Autodesk Fusion 360 part; units mm, degrees
note: some values were not read from the file. Set by a fixed rule: which sketch regions a step uses.
(part 2 of 4)
  spline S190 degree 3 poles (159.041, -110.49) (158.9881, -111.6013) (157.4271, -114.2471) (156.1835, -115.2525) knots 0 0 0 0 1 1 1 1
  spline S191 degree 3 poles (156.1835, -115.2525) (154.7283, -116.4431) (153.0085, -116.9458) (150.3892, -116.9458) knots 0 0 0 0 1 1 1 1
  spline S192 degree 3 poles (150.3892, -116.9458) (148.9604, -116.9458) (148.3519, -117.0517) (147.9285, -117.3956) knots 0 0 0 0 1 1 1 1
  line L118 (147.9285, -117.3956) -> (147.3465, -117.8719)
  line L119 (147.3465, -117.8719) -> (147.9021, -119.4594)
  spline S193 degree 3 poles (147.9021, -119.4594) (148.881, -122.211) (149.2779, -124.8304) (149.2515, -128.4552) knots 0 0 0 0 1 1 1 1
  spline S194 degree 3 poles (149.2515, -128.4552) (149.2515, -132.5298) (148.5635, -135.7048) (146.8967, -139.2502) knots 0 0 0 0 1 1 1 1
  line L120 (146.8967, -139.2502) -> (145.8648, -141.4727)
  line L121 (145.8648, -141.4727) -> (146.9496, -141.2346)
  spline S195 degree 3 poles (146.9496, -141.2346) (147.5317, -141.0758) (149.0133, -141.0229) (150.2304, -141.1023) knots 0 0 0 0 1 1 1 1
  spline S196 degree 3 poles (150.2304, -141.1023) (153.035, -141.261) (155.1781, -142.2135) (155.7338, -143.5629) knots 0 0 0 0 1 1 1 1
  spline S197 degree 3 poles (155.7338, -143.5629) (156.2365, -144.7271) (156.21, -147.8227) (155.6808, -151.2094) knots 0 0 0 0 1 1 1 1
  spline S198 degree 3 poles (155.6808, -151.2094) (155.231, -154.1462) (155.284, -154.7813) (156.0248, -154.7813) knots 0 0 0 0 1 1 1 1
  spline S199 degree 3 poles (156.0248, -154.7813) (157.136, -154.7813) (158.1944, -153.7494) (159.1469, -151.765) knots 0 0 0 0 1 1 1 1
  spline S200 degree 3 poles (159.1469, -151.765) (160.1258, -149.7013) (160.7344, -149.1192) (161.7398, -149.2779) knots 0 0 0 0 1 1 1 1
  spline S201 degree 3 poles (161.7398, -149.2779) (162.6658, -149.4102) (162.6394, -150.5479) (161.6604, -151.474) knots 0 0 0 0 1 1 1 1
  spline S202 degree 3 poles (161.6604, -151.474) (160.7873, -152.2942) (160.6021, -153.1938) (161.3165, -153.1938) knots 0 0 0 0 1 1 1 1
  spline S203 degree 3 poles (161.3165, -153.1938) (161.5546, -153.1938) (162.5071, -152.9027) (163.4067, -152.5323) knots 0 0 0 0 1 1 1 1
  spline S204 degree 3 poles (163.4067, -152.5323) (164.9677, -151.8973) (167.0315, -151.6063) (167.3754, -151.9502) knots 0 0 0 0 1 1 1 1
  spline S205 degree 3 poles (167.3754, -151.9502) (167.8252, -152.3735) (167.1108, -153.1938) (166.079, -153.4583) knots 0 0 0 0 1 1 1 1
  spline S206 degree 3 poles (166.079, -153.4583) (164.5708, -153.8288) (162.56, -154.8606) (162.7188, -155.1781) knots 0 0 0 0 1 1 1 1
  spline S207 degree 3 poles (162.7188, -155.1781) (162.7981, -155.3104) (163.0363, -155.4163) (163.2479, -155.3633) knots 0 0 0 0 1 1 1 1
  spline S208 degree 3 poles (163.2479, -155.3633) (164.9942, -154.9929) (166.661, -154.8077) (168.8835, -154.8077) knots 0 0 0 0 1 1 1 1
  spline S209 degree 3 poles (168.8835, -154.8077) (171.3971, -154.7813) (171.4765, -154.8077) (171.3971, -155.3633) knots 0 0 0 0 1 1 1 1
  spline S210 degree 3 poles (171.3971, -155.3633) (171.3177, -155.9983) (170.9473, -156.1306) (168.1427, -156.6333) knots 0 0 0 0 1 1 1 1
  spline S211 degree 3 poles (168.1427, -156.6333) (165.7615, -157.0831) (163.7771, -157.6652) (163.7771, -157.9298) knots 0 0 0 0 1 1 1 1
  spline S212 degree 3 poles (163.7771, -157.9298) (163.7771, -158.2738) (166.37, -159.0146) (169.0158, -159.4115) knots 0 0 0 0 1 1 1 1
  spline S213 degree 3 poles (169.0158, -159.4115) (171.7675, -159.8348) (171.9792, -159.9142) (171.9792, -160.5756) knots 0 0 0 0 1 1 1 1
  spline S214 degree 3 poles (171.9792, -160.5756) (171.9792, -161.7663) (171.0267, -161.925) (168.1956, -161.1048) knots 0 0 0 0 1 1 1 1
  spline S215 degree 3 poles (168.1956, -161.1048) (167.1638, -160.8138) (165.1529, -160.5227) (163.7771, -160.4433) knots 0 0 0 0 1 1 1 1
  spline S216 degree 3 poles (163.7771, -160.4433) (161.581, -160.311) (161.3165, -160.3375) (161.7398, -160.6815) knots 0 0 0 0 1 1 1 1
  spline S217 degree 3 poles (161.7398, -160.6815) (161.9779, -160.8931) (162.7981, -161.1313) (163.539, -161.2106) knots 0 0 0 0 1 1 1 1
  spline S218 degree 3 poles (163.539, -161.2106) (165.1, -161.3958) (165.6821, -161.7927) (165.5763, -162.56) knots 0 0 0 0 1 1 1 1
  spline S219 degree 3 poles (165.5763, -162.56) (165.4969, -163.0627) (165.3381, -163.1156) (164.0417, -163.0892) knots 0 0 0 0 1 1 1 1
  spline S220 degree 3 poles (164.0417, -163.0892) (163.2479, -163.0627) (161.925, -162.7981) (161.1313, -162.5071) knots 0 0 0 0 1 1 1 1
  spline S221 degree 3 poles (161.1313, -162.5071) (154.1992, -159.9406) (153.67, -159.7025) (152.4529, -158.459) knots 0 0 0 0 1 1 1 1
  spline S222 degree 3 poles (152.4529, -158.459) (151.0506, -157.0302) (150.0188, -153.4848) (150.0188, -150.0452) knots 0 0 0 0 1 1 1 1
  spline S223 degree 3 poles (150.0188, -150.0452) (150.0188, -148.8017) (149.9658, -148.6694) (149.569, -148.8546) knots 0 0 0 0 1 1 1 1
  spline S224 degree 3 poles (149.569, -148.8546) (148.6694, -149.225) (145.6531, -149.9923) (144.9388, -149.9923) knots 0 0 0 0 1 1 1 1
  spline S225 degree 3 poles (144.9388, -149.9923) (144.1979, -150.0188) (144.1979, -150.0188) (144.1979, -151.8708) knots 0 0 0 0 1 1 1 1
  spline S226 degree 3 poles (144.1979, -151.8708) (144.1979, -154.305) (143.51, -156.3158) (141.5521, -159.676) knots 0 0 0 0 1 1 1 1
  spline S227 degree 3 poles (141.5521, -159.676) (138.5888, -164.809) (137.1335, -169.201) (136.869, -173.8313) knots 0 0 0 0 1 1 1 1
  spline S228 degree 3 poles (136.869, -173.8313) (136.4985, -181.1073) (139.5677, -185.42) (147.664, -189.0183) knots 0 0 0 0 1 1 1 1
  spline S229 degree 3 poles (147.664, -189.0183) (151.13, -190.5529) (157.4271, -191.0292) (162.0044, -190.0767) knots 0 0 0 0 1 1 1 1
  spline S230 degree 3 poles (162.0044, -190.0767) (169.7038, -188.5156) (175.8685, -184.6792) (181.4777, -177.9323) knots 0 0 0 0 1 1 1 1
  line L122 (181.4777, -177.9323) -> (182.3508, -176.874)
  line L123 (182.3508, -176.874) -> (181.6629, -178.1969)
  spline S231 degree 3 poles (181.6629, -178.1969) (178.4879, -184.2029) (172.1379, -189.1242) (164.0417, -191.8494) knots 0 0 0 0 1 1 1 1
  spline S232 degree 3 poles (164.0417, -191.8494) (155.1252, -194.8392) (147.0025, -194.7863) (139.6735, -191.6906) knots 0 0 0 0 1 1 1 1
  spline S233 degree 3 poles (139.6735, -191.6906) (127.344, -186.5048) (124.5658, -178.2233) (130.0163, -163.0627) knots 0 0 0 0 1 1 1 1
  spline S234 degree 3 poles (130.0163, -163.0627) (131.2333, -159.7025) (131.4979, -156.9773) (130.8894, -153.8552) knots 0 0 0 0 1 1 1 1
  spline S235 degree 3 poles (130.8894, -153.8552) (130.3338, -150.8919) (130.0427, -150.3098) (129.0638, -149.8865) knots 0 0 0 0 1 1 1 1
  spline S236 degree 3 poles (129.0638, -149.8865) (128.5875, -149.7013) (127.6615, -149.1192) (127, -148.6165) knots 0 0 0 0 1 1 1 1
  line L124 (127, -148.6165) -> (125.8094, -147.7169)
  line L125 (125.8094, -147.7169) -> (125.8094, -150.6538)
  spline S237 degree 3 poles (125.8094, -150.6538) (125.8094, -153.4319) (125.7565, -153.6965) (124.9627, -155.3104) knots 0 0 0 0 1 1 1 1
  spline S238 degree 3 poles (124.9627, -155.3104) (123.825, -157.6388) (123.0577, -158.3002) (119.8298, -159.7025) knots 0 0 0 0 1 1 1 1
  spline S239 degree 3 poles (119.8298, -159.7025) (113.1623, -162.6394) (110.834, -163.2479) (110.0667, -162.2954) knots 0 0 0 0 1 1 1 1
  spline S240 degree 3 poles (110.0667, -162.2954) (109.564, -161.7398) (110.1196, -161.29) (111.7865, -160.8931) knots 0 0 0 0 1 1 1 1
  spline S241 degree 3 poles (111.7865, -160.8931) (112.5273, -160.7079) (113.5063, -160.311) (113.9825, -160.02) knots 0 0 0 0 1 1 1 1
  spline S242 degree 3 poles (113.9825, -160.02) (114.7233, -159.5702) (114.8027, -159.4379) (114.5117, -159.094) knots 0 0 0 0 1 1 1 1
  spline S243 degree 3 poles (114.5117, -159.094) (114.2471, -158.75) (113.7444, -158.7235) (111.6542, -158.8558) knots 0 0 0 0 1 1 1 1
  spline S244 degree 3 poles (111.6542, -158.8558) (105.1454, -159.3056) (104.0871, -159.3321) (103.3992, -159.041) knots 0 0 0 0 1 1 1 1
  spline S245 degree 3 poles (103.3992, -159.041) (102.6319, -158.75) (102.3938, -158.0356) (103.0023, -157.824) knots 0 0 0 0 1 1 1 1
  spline S246 degree 3 poles (103.0023, -157.824) (103.161, -157.771) (104.9338, -157.5858) (106.8917, -157.4535) knots 0 0 0 0 1 1 1 1
  spline S247 degree 3 poles (106.8917, -157.4535) (110.9663, -157.1625) (112.4479, -156.7921) (111.8658, -156.1835) knots 0 0 0 0 1 1 1 1
  spline S248 degree 3 poles (111.8658, -156.1835) (111.6542, -155.9983) (111.0192, -155.7602) (110.4371, -155.6808) knots 0 0 0 0 1 1 1 1
  spline S249 degree 3 poles (110.4371, -155.6808) (108.876, -155.4427) (104.5898, -154.014) (104.2458, -153.5906) knots 0 0 0 0 1 1 1 1
  spline S250 degree 3 poles (104.2458, -153.5906) (104.0606, -153.379) (104.0077, -153.0085) (104.0871, -152.7704) knots 0 0 0 0 1 1 1 1
  spline S251 degree 3 poles (104.0871, -152.7704) (104.2988, -152.2413) (105.5158, -152.3735) (109.2729, -153.3525) knots 0 0 0 0 1 1 1 1
  spline S252 degree 3 poles (109.2729, -153.3525) (112.1304, -154.0669) (112.7125, -154.1198) (112.7125, -153.6435) knots 0 0 0 0 1 1 1 1
  spline S253 degree 3 poles (112.7125, -153.6435) (112.7125, -153.1938) (111.76, -152.2942) (110.146, -151.2358) knots 0 0 0 0 1 1 1 1
  spline S254 degree 3 poles (110.146, -151.2358) (108.876, -150.4156) (108.4527, -149.6748) (108.9554, -149.1721) knots 0 0 0 0 1 1 1 1
  spline S255 degree 3 poles (108.9554, -149.1721) (109.4317, -148.6958) (110.781, -149.225) (112.6067, -150.5744) knots 0 0 0 0 1 1 1 1
  spline S256 degree 3 poles (112.6067, -150.5744) (113.5856, -151.2887) (114.4852, -151.8708) (114.591, -151.8708) knots 0 0 0 0 1 1 1 1
  spline S257 degree 3 poles (114.591, -151.8708) (114.9879, -151.8708) (114.8556, -150.839) (114.3, -149.7542) knots 0 0 0 0 1 1 1 1
  spline S258 degree 3 poles (114.3, -149.7542) (113.6121, -148.4048) (113.6121, -147.2142) (114.2735, -147.029) knots 0 0 0 0 1 1 1 1
  spline S259 degree 3 poles (114.2735, -147.029) (114.9879, -146.8438) (115.8875, -147.5317) (115.8875, -148.246) knots 0 0 0 0 1 1 1 1
  spline S260 degree 3 poles (115.8875, -148.246) (115.8875, -149.3044) (118.2158, -152.2413) (119.38, -152.6381) knots 0 0 0 0 1 1 1 1
  spline S261 degree 3 poles (119.38, -152.6381) (120.2002, -152.9292) (120.9146, -152.7704) (120.9146, -152.2942) knots 0 0 0 0 1 1 1 1
  spline S262 degree 3 poles (120.9146, -152.2942) (120.9146, -152.1354) (120.6765, -151.1035) (120.3854, -150.0188) knots 0 0 0 0 1 1 1 1
  spline S263 degree 3 poles (120.3854, -150.0188) (119.4858, -146.6056) (119.8563, -143.3248) (121.3115, -141.605) knots 0 0 0 0 1 1 1 1
  spline S264 degree 3 poles (121.3115, -141.605) (122.1581, -140.5996) (122.9783, -140.4408) (125.5448, -140.9171) knots 0 0 0 0 1 1 1 1
  spline S265 degree 3 poles (125.5448, -140.9171) (126.709, -141.1023) (127.926, -141.2875) (128.2435, -141.2875) knots 0 0 0 0 1 1 1 1
  line L126 (128.2435, -141.2875) -> (128.8256, -141.2875)
  line L127 (128.8256, -141.2875) -> (128.0054, -139.0915)
  spline S266 degree 3 poles (128.0054, -139.0915) (125.3596, -132.08) (124.5129, -127.8202) (124.6981, -122.5021) knots 0 0 0 0 1 1 1 1
  spline S267 degree 3 poles (124.6981, -122.5021) (124.8304, -119.1948) (125.1479, -117.5015) (126.0475, -115.3319) knots 0 0 0 0 1 1 1 1
  spline S268 degree 3 poles (126.0475, -115.3319) (126.3385, -114.6704) (124.9363, -114.3) (122.2375, -114.3) knots 0 0 0 0 1 1 1 1
  spline S269 degree 3 poles (122.2375, -114.3) (120.1473, -114.3) (119.8563, -114.2206) (118.6392, -113.4798) knots 0 0 0 0 1 1 1 1
  spline S270 degree 3 poles (118.6392, -113.4798) (117.9248, -113.03) (116.9988, -112.3421) (116.5754, -111.9452) knots 0 0 0 0 1 1 1 1
  spline S271 degree 3 poles (116.5754, -111.9452) (115.7817, -111.2308) (114.5646, -108.929) (114.5646, -108.1881) knots 0 0 0 0 1 1 1 1
  spline S272 degree 3 poles (114.5646, -108.1881) (114.5646, -107.7383) (113.321, -106.4948) (112.051, -105.6746) knots 0 0 0 0 1 1 1 1
  spline S273 degree 3 poles (112.051, -105.6746) (111.7071, -105.4365) (110.9398, -105.1983) (110.3313, -105.1454) knots 0 0 0 0 1 1 1 1
  spline S274 degree 3 poles (110.3313, -105.1454) (108.8496, -105.0131) (106.5742, -103.8225) (106.68, -103.2404) knots 0 0 0 0 1 1 1 1
  spline S275 degree 3 poles (106.68, -103.2404) (106.7858, -102.7906) (107.4473, -102.7112) (109.0083, -102.9494) knots 0 0 0 0 1 1 1 1
  spline S276 degree 3 poles (109.0083, -102.9494) (109.511, -103.0288) (109.6963, -102.9229) (109.7492, -102.526) knots 0 0 0 0 1 1 1 1
  spline S277 degree 3 poles (109.7492, -102.526) (109.8021, -102.1556) (108.9819, -101.1502) (107.1563, -99.2981) knots 0 0 0 0 1 1 1 1
  spline S278 degree 3 poles (107.1563, -99.2981) (105.701, -97.8165) (104.5104, -96.4671) (104.5104, -96.3083) knots 0 0 0 0 1 1 1 1
  spline S279 degree 3 poles (104.5104, -96.3083) (104.5104, -95.8585) (105.754, -95.6998) (106.7329, -96.0438) knots 0 0 0 0 1 1 1 1
  spline S280 degree 3 poles (106.7329, -96.0438) (107.315, -96.229) (108.0558, -96.8375) (108.6644, -97.5783) knots 0 0 0 0 1 1 1 1
  spline S281 degree 3 poles (108.6644, -97.5783) (109.22, -98.2662) (109.8021, -98.9012) (109.9344, -99.0071) knots 0 0 0 0 1 1 1 1
  spline S282 degree 3 poles (109.9344, -99.0071) (110.834, -99.6685) (110.8075, -98.6102) (109.8815, -96.7317) knots 0 0 0 0 1 1 1 1
  spline S283 degree 3 poles (109.8815, -96.7317) (109.1671, -95.2235) (109.1935, -94.4563) (110.0138, -94.4563) knots 0 0 0 0 1 1 1 1
  spline S284 degree 3 poles (110.0138, -94.4563) (110.7017, -94.4563) (111.4954, -95.4087) (112.2892, -97.155) knots 0 0 0 0 1 1 1 1
  spline S285 degree 3 poles (112.2892, -97.155) (113.321, -99.5362) (114.0354, -99.0865) (114.0354, -96.0967) knots 0 0 0 0 1 1 1 1
  spline S286 degree 3 poles (114.0354, -96.0967) (114.0354, -94.959) (114.1677, -94.5621) (114.7233, -94.0065) knots 0 0 0 0 1 1 1 1
  spline S287 degree 3 poles (114.7233, -94.0065) (115.3319, -93.3979) (115.4377, -93.3715) (115.8081, -93.7154) knots 0 0 0 0 1 1 1 1
  spline S288 degree 3 poles (115.8081, -93.7154) (116.1256, -94.0594) (116.1521, -94.324) (115.914, -95.1442) knots 0 0 0 0 1 1 1 1
  spline S289 degree 3 poles (115.914, -95.1442) (115.5435, -96.4671) (115.5435, -98.5837) (115.8875, -99.2452) knots 0 0 0 0 1 1 1 1
  spline S290 degree 3 poles (115.8875, -99.2452) (116.3902, -100.1712) (117.1575, -99.8538) (117.8719, -98.425) knots 0 0 0 0 1 1 1 1
  spline S291 degree 3 poles (117.8719, -98.425) (118.3481, -97.4725) (118.6921, -97.1021) (119.089, -97.1021) knots 0 0 0 0 1 1 1 1
  spline S292 degree 3 poles (119.089, -97.1021) (119.7504, -97.1021) (119.671, -97.3931) (118.3481, -100.3829) knots 0 0 0 0 1 1 1 1
  spline S293 degree 3 poles (118.3481, -100.3829) (117.3427, -102.6054) (117.0517, -104.0606) (117.3163, -105.1719) knots 0 0 0 0 1 1 1 1
  spline S294 degree 3 poles (117.3163, -105.1719) (117.5015, -105.9392) (118.9302, -107.5796) (120.3854, -108.7438) knots 0 0 0 0 1 1 1 1
  line L128 (120.3854, -108.7438) -> (121.3644, -109.511)
  line L129 (121.3644, -109.511) -> (123.4281, -108.8496)
  spline S295 degree 3 poles (123.4281, -108.8496) (124.751, -108.4262) (126.1533, -108.1881) (127.3704, -108.1617) knots 0 0 0 0 1 1 1 1
  line L130 (127.3704, -108.1617) -> (129.249, -108.1352)
  line L131 (129.249, -108.1352) -> (130.4131, -106.68)
  spline S296 degree 3 poles (130.4131, -106.68) (131.736, -105.0131) (132.1858, -103.7167) (131.7625, -102.9229) knots 0 0 0 0 1 1 1 1
  spline S297 degree 3 poles (131.7625, -102.9229) (131.6038, -102.6319) (131.3921, -102.3938) (131.2598, -102.3938) knots 0 0 0 0 1 1 1 1
  spline S298 degree 3 poles (131.2598, -102.3938) (130.7571, -102.3938) (129.1167, -100.3829) (128.7463, -99.2717) knots 0 0 0 0 1 1 1 1
  spline S299 degree 3 poles (128.7463, -99.2717) (128.27, -97.8958) (128.1906, -94.0594) (128.5875, -92.5777) knots 0 0 0 0 1 1 1 1
  spline S300 degree 3 poles (128.5875, -92.5777) (128.7463, -92.0485) (129.1431, -91.2019) (129.5135, -90.7256) knots 0 0 0 0 1 1 1 1
  spline S301 degree 3 poles (129.5135, -90.7256) (129.8575, -90.2229) (130.3338, -89.4292) (130.5454, -88.9794) knots 0 0 0 0 1 1 1 1
  spline S302 degree 3 poles (130.5454, -88.9794) (130.7571, -88.5031) (131.2863, -87.6035) (131.7096, -86.995) knots 0 0 0 0 1 1 1 1
  spline S303 degree 3 poles (131.7096, -86.995) (132.1329, -86.36) (132.8473, -85.09) (133.2706, -84.1375) knots 0 0 0 0 1 1 1 1
  spline S304 degree 3 poles (133.2706, -84.1375) (134.1173, -82.259) (135.4138, -80.645) (136.6573, -79.8512) knots 0 0 0 0 1 1 1 1
  spline S305 degree 3 poles (136.6573, -79.8512) (137.7156, -79.1633) (140.679, -79.3221) (142.24, -80.1158) knots 0 0 0 0 1 1 1 1
  spline S306 degree 3 poles (215.6354, -67.7598) (211.0581, -70.9612) (207.2217, -73.66) (207.0894, -73.7923) knots 0 0 0 0 1 1 1 1
  spline S307 degree 3 poles (207.0894, -73.7923) (206.8248, -74.0569) (213.6775, -84.164) (216.8525, -88.265) knots 0 0 0 0 1 1 1 1
  spline S308 degree 3 poles (216.8525, -88.265) (219.0221, -91.0696) (221.4298, -93.2127) (223.5729, -94.271) knots 0 0 0 0 1 1 1 1
  spline S309 degree 3 poles (223.5729, -94.271) (224.9752, -94.959) (225.6102, -95.1177) (227.039, -95.1177) knots 0 0 0 0 1 1 1 1
  spline S310 degree 3 poles (227.039, -95.1177) (228.5471, -95.1177) (229.0498, -94.9854) (230.796, -94.0858) knots 0 0 0 0 1 1 1 1
  spline S311 degree 3 poles (230.796, -94.0858) (233.389, -92.7894) (235.9025, -90.514) (236.6963, -88.7677) knots 0 0 0 0 1 1 1 1
  spline S312 degree 3 poles (236.6963, -88.7677) (237.9398, -86.1219) (237.3577, -82.4442) (235.0294, -78.0521) knots 0 0 0 0 1 1 1 1
  spline S313 degree 3 poles (235.0294, -78.0521) (233.8917, -75.909) (224.3931, -61.886) (224.1021, -61.939) knots 0 0 0 0 1 1 1 1
  spline S314 degree 3 poles (224.1021, -61.939) (224.0227, -61.939) (220.2127, -64.5848) (215.6354, -67.7598) knots 0 0 0 0 1 1 1 1
  spline S315 degree 3 poles (227.0654, -75.0358) (231.0606, -80.8567) (230.9283, -83.82) (226.5627, -86.069) knots 0 0 0 0 1 1 1 1
  spline S316 degree 3 poles (226.5627, -86.069) (224.6842, -87.0479) (222.2765, -86.3335) (220.3715, -84.2433) knots 0 0 0 0 1 1 1 1
  spline S317 degree 3 poles (220.3715, -84.2433) (219.3131, -83.0792) (216.1381, -78.5283) (216.2175, -78.2638) knots 0 0 0 0 1 1 1 1
  spline S318 degree 3 poles (216.2175, -78.2638) (216.3498, -77.8933) (224.7106, -72.2048) (225.0017, -72.3106) knots 0 0 0 0 1 1 1 1
  spline S319 degree 3 poles (225.0017, -72.3106) (225.134, -72.3635) (226.06, -73.5806) (227.0654, -75.0358) knots 0 0 0 0 1 1 1 1
  spline S320 degree 3 poles (57.5469, -81.1212) (55.245, -84.6931) (53.2606, -87.6565) (53.1283, -87.7358) knots 0 0 0 0 1 1 1 1
  spline S321 degree 3 poles (53.1283, -87.7358) (52.996, -87.8152) (49.9269, -85.9367) (46.2756, -83.5819) knots 0 0 0 0 1 1 1 1
  spline S322 degree 3 poles (46.2756, -83.5819) (42.6508, -81.2271) (39.5552, -79.4015) (39.4494, -79.5337) knots 0 0 0 0 1 1 1 1
  spline S323 degree 3 poles (39.4494, -79.5337) (38.4969, -80.6715) (34.8985, -86.5981) (35.0838, -86.7833) knots 0 0 0 0 1 1 1 1
  spline S324 degree 3 poles (35.0838, -86.7833) (35.4542, -87.1273) (52.1494, -97.9223) (52.414, -97.9752) knots 0 0 0 0 1 1 1 1
  spline S325 degree 3 poles (52.414, -97.9752) (52.5727, -98.0017) (55.6948, -93.3979) (59.3725, -87.7094) knots 0 0 0 0 1 1 1 1
  line L132 (59.3725, -87.7094) -> (66.0929, -77.3906)
  line L133 (66.0929, -77.3906) -> (64.1879, -76.2)
  spline S326 degree 3 poles (64.1879, -76.2) (63.156, -75.5385) (62.1771, -74.9035) (62.0183, -74.7977) knots 0 0 0 0 1 1 1 1
  spline S327 degree 3 poles (62.0183, -74.7977) (61.8596, -74.7183) (60.034, -77.2583) (57.5469, -81.1212) knots 0 0 0 0 1 1 1 1
  spline S328 degree 3 poles (188.7538, -117.184) (186.9546, -118.0042) (186.2667, -120.2002) (187.325, -121.8935) knots 0 0 0 0 1 1 1 1
  spline S329 degree 3 poles (187.325, -121.8935) (188.7538, -124.2483) (192.2727, -124.0102) (193.331, -121.5231) knots 0 0 0 0 1 1 1 1
  spline S330 degree 3 poles (193.331, -121.5231) (194.0719, -119.6975) (193.2781, -117.8454) (191.3731, -117.0517) knots 0 0 0 0 1 1 1 1
  spline S331 degree 3 poles (191.3731, -117.0517) (190.2883, -116.5754) (190.0502, -116.6019) (188.7538, -117.184) knots 0 0 0 0 1 1 1 1
  spline S332 degree 3 poles (81.3329, -117.9777) (80.2217, -118.4804) (79.375, -119.7504) (79.375, -120.8881) knots 0 0 0 0 1 1 1 1
  spline S333 degree 3 poles (79.375, -120.8881) (79.375, -122.6608) (81.0154, -124.3542) (82.7617, -124.3542) knots 0 0 0 0 1 1 1 1
  spline S334 degree 3 poles (82.7617, -124.3542) (86.3865, -124.3542) (87.5506, -119.4594) (84.2963, -117.9777) knots 0 0 0 0 1 1 1 1
  spline S335 degree 3 poles (84.2963, -117.9777) (83.6877, -117.7131) (83.0263, -117.475) (82.8146, -117.475) knots 0 0 0 0 1 1 1 1
  spline S336 degree 3 poles (82.8146, -117.475) (82.6029, -117.475) (81.9415, -117.7131) (81.3329, -117.9777) knots 0 0 0 0 1 1 1 1
  spline S337 degree 3 poles (200.3954, -129.9104) (200.1044, -130.0163) (199.5223, -130.4925) (199.1519, -130.9688) knots 0 0 0 0 1 1 1 1
  spline S338 degree 3 poles (199.1519, -130.9688) (197.776, -132.5827) (198.3317, -135.1227) (200.2896, -136.1281) knots 0 0 0 0 1 1 1 1
  spline S339 degree 3 poles (200.2896, -136.1281) (202.5121, -137.2658) (205.0521, -135.6254) (205.0521, -133.0854) knots 0 0 0 0 1 1 1 1
  spline S340 degree 3 poles (205.0521, -133.0854) (205.0521, -130.6513) (202.6444, -128.9844) (200.3954, -129.9104) knots 0 0 0 0 1 1 1 1
  spline S341 degree 3 poles (92.366, -132.715) (91.1754, -133.7204) (90.8579, -135.1492) (91.5194, -136.6308) knots 0 0 0 0 1 1 1 1
  spline S342 degree 3 poles (91.5194, -136.6308) (92.9746, -139.9381) (97.8958, -138.9592) (97.8958, -135.3344) knots 0 0 0 0 1 1 1 1
  spline S343 degree 3 poles (97.8958, -135.3344) (97.8958, -133.2706) (96.5465, -132.0271) (94.3504, -132.0271) knots 0 0 0 0 1 1 1 1
  spline S344 degree 3 poles (94.3504, -132.0271) (93.4773, -132.0271) (92.9746, -132.1858) (92.366, -132.715) knots 0 0 0 0 1 1 1 1
  spline S345 degree 3 poles (180.049, -136.9748) (178.5144, -137.3717) (177.5354, -138.7475) (177.5354, -140.4938) knots 0 0 0 0 1 1 1 1
  spline S346 degree 3 poles (177.5354, -140.4938) (177.5354, -142.0019) (178.8054, -143.3777) (180.3665, -143.5894) knots 0 0 0 0 1 1 1 1
  spline S347 degree 3 poles (180.3665, -143.5894) (182.4038, -143.854) (183.9119, -142.7427) (184.2558, -140.7583) knots 0 0 0 0 1 1 1 1
  spline S348 degree 3 poles (184.2558, -140.7583) (184.6527, -138.5888) (182.2185, -136.4192) (180.049, -136.9748) knots 0 0 0 0 1 1 1 1
  spline S349 degree 3 poles (71.411, -140.2027) (70.5379, -141.0758) (70.3792, -141.3933) (70.3792, -142.3723) knots 0 0 0 0 1 1 1 1
  spline S350 degree 3 poles (70.3792, -142.3723) (70.3792, -145.4679) (73.6071, -147.0554) (75.909, -145.0975) knots 0 0 0 0 1 1 1 1
  spline S351 degree 3 poles (75.909, -145.0975) (77.2319, -144.0127) (77.4435, -142.2929) (76.491, -140.5202) knots 0 0 0 0 1 1 1 1
  spline S352 degree 3 poles (76.491, -140.5202) (76.0677, -139.7529) (74.8242, -139.1708) (73.5277, -139.1708) knots 0 0 0 0 1 1 1 1
  spline S353 degree 3 poles (73.5277, -139.1708) (72.6017, -139.1708) (72.2577, -139.3296) (71.411, -140.2027) knots 0 0 0 0 1 1 1 1
  spline S354 degree 3 poles (190.6588, -151.8973) (187.9865, -153.9875) (189.2829, -157.9563) (192.6167, -157.9563) knots 0 0 0 0 1 1 1 1
  spline S355 degree 3 poles (192.6167, -157.9563) (194.019, -157.9563) (195.0244, -157.3477) (195.6594, -156.1042) knots 0 0 0 0 1 1 1 1
  spline S356 degree 3 poles (195.6594, -156.1042) (196.7971, -153.8817) (195.1567, -151.3417) (192.6167, -151.3417) knots 0 0 0 0 1 1 1 1
  spline S357 degree 3 poles (192.6167, -151.3417) (191.7435, -151.3417) (191.1615, -151.5004) (190.6588, -151.8973) knots 0 0 0 0 1 1 1 1
  spline S358 degree 3 poles (83.1056, -152.7969) (82.0473, -153.7229) (81.5975, -155.0723) (81.9944, -156.3423) knots 0 0 0 0 1 1 1 1
  spline S359 degree 3 poles (81.9944, -156.3423) (82.4442, -157.8504) (83.3438, -158.5648) (85.0371, -158.6971) knots 0 0 0 0 1 1 1 1
  spline S360 degree 3 poles (85.0371, -158.6971) (86.36, -158.8029) (86.5188, -158.75) (87.4713, -157.8769) knots 0 0 0 0 1 1 1 1
  spline S361 degree 3 poles (87.4713, -157.8769) (88.4238, -157.0038) (88.5031, -156.845) (88.5031, -155.4427) knots 0 0 0 0 1 1 1 1
  spline S362 degree 3 poles (88.5031, -155.4427) (88.5031, -154.0404) (88.4238, -153.8817) (87.5242, -153.035) knots 0 0 0 0 1 1 1 1
  spline S363 degree 3 poles (87.5242, -153.035) (86.6775, -152.2677) (86.3335, -152.1354) (85.2223, -152.1354) knots 0 0 0 0 1 1 1 1
  spline S364 degree 3 poles (85.2223, -152.1354) (84.2169, -152.1354) (83.7406, -152.2942) (83.1056, -152.7969) knots 0 0 0 0 1 1 1 1
  spline S365 degree 3 poles (34.1048, -156.501) (29.8185, -157.6917) (26.1673, -158.7235) (26.035, -158.7765) knots 0 0 0 0 1 1 1 1
  spline S366 degree 3 poles (26.035, -158.7765) (25.8233, -158.8558) (30.9563, -178.435) (31.2738, -178.7525) knots 0 0 0 0 1 1 1 1
  spline S367 degree 3 poles (31.2738, -178.7525) (31.3796, -178.8319) (34.9515, -177.8529) (35.1102, -177.6942) knots 0 0 0 0 1 1 1 1
  spline S368 degree 3 poles (35.1102, -177.6942) (35.1631, -177.6413) (34.4223, -174.7308) (33.4698, -171.1854) knots 0 0 0 0 1 1 1 1
  spline S369 degree 3 poles (33.4698, -171.1854) (32.4908, -167.6665) (31.75, -164.7296) (31.8294, -164.6767) knots 0 0 0 0 1 1 1 1
  spline S370 degree 3 poles (31.8294, -164.6767) (31.9088, -164.5973) (32.4908, -164.3592) (33.1523, -164.174) knots 0 0 0 0 1 1 1 1
  line L134 (33.1523, -164.174) -> (34.3694, -163.8035)
  line L135 (34.3694, -163.8035) -> (34.7663, -165.1794)
  spline S371 degree 3 poles (34.7663, -165.1794) (34.9779, -165.9467) (35.5865, -168.1692) (36.1421, -170.1271) knots 0 0 0 0 1 1 1 1
  spline S372 degree 3 poles (36.1421, -170.1271) (36.6713, -172.085) (37.2004, -173.8048) (37.3063, -173.9106) knots 0 0 0 0 1 1 1 1
  spline S373 degree 3 poles (37.3063, -173.9106) (37.4915, -174.1223) (39.6081, -173.646) (40.0315, -173.3021) knots 0 0 0 0 1 1 1 1
  spline S374 degree 3 poles (40.0315, -173.3021) (40.1638, -173.1962) (39.6346, -170.8679) (38.8938, -168.1427) knots 0 0 0 0 1 1 1 1
  spline S375 degree 3 poles (38.8938, -168.1427) (38.1529, -165.4175) (37.5973, -163.1421) (37.6502, -163.0627) knots 0 0 0 0 1 1 1 1
  spline S376 degree 3 poles (37.6502, -163.0627) (37.7296, -163.0098) (38.3381, -162.7717) (38.9996, -162.5865) knots 0 0 0 0 1 1 1 1
  spline S377 degree 3 poles (38.9996, -162.5865) (39.9521, -162.2954) (40.2696, -162.269) (40.349, -162.5335) knots 0 0 0 0 1 1 1 1
  spline S378 degree 3 poles (40.349, -162.5335) (40.4019, -162.7188) (41.1427, -165.3381) (41.9629, -168.4073) knots 0 0 0 0 1 1 1 1
  spline S379 degree 3 poles (41.9629, -168.4073) (42.7831, -171.45) (43.5504, -174.0694) (43.6563, -174.1752) knots 0 0 0 0 1 1 1 1
  spline S380 degree 3 poles (43.6563, -174.1752) (43.9473, -174.5192) (47.4927, -173.4344) (47.4663, -173.011) knots 0 0 0 0 1 1 1 1
  spline S381 degree 3 poles (47.4663, -173.011) (47.4398, -172.6406) (43.8415, -159.5438) (42.836, -156.0248) knots 0 0 0 0 1 1 1 1
  spline S382 degree 3 poles (42.836, -156.0248) (42.545, -155.0458) (42.2275, -154.2521) (42.1217, -154.2785) knots 0 0 0 0 1 1 1 1
  spline S383 degree 3 poles (42.1217, -154.2785) (42.0158, -154.305) (38.4175, -155.284) (34.1048, -156.501) knots 0 0 0 0 1 1 1 1
  spline S384 degree 3 poles (236.0083, -155.2046) (232.7804, -156.5804) (230.1346, -162.2425) (230.0817, -167.8781) knots 0 0 0 0 1 1 1 1
  spline S385 degree 3 poles (230.0817, -167.8781) (230.0552, -170.3388) (230.1081, -170.6298) (230.8225, -171.9262) knots 0 0 0 0 1 1 1 1
  spline S386 degree 3 poles (230.8225, -171.9262) (232.119, -174.2281) (234.1298, -175.3923) (236.0083, -174.8896) knots 0 0 0 0 1 1 1 1
  spline S387 degree 3 poles (236.0083, -174.8896) (237.8869, -174.3869) (239.2892, -172.2438) (241.1677, -166.9521) knots 0 0 0 0 1 1 1 1
  spline S388 degree 3 poles (241.1677, -166.9521) (242.5171, -163.1421) (242.861, -162.7717) (243.5754, -164.4385) knots 0 0 0 0 1 1 1 1
  spline S389 degree 3 poles (243.5754, -164.4385) (244.1046, -165.7085) (243.6813, -167.296) (242.4906, -168.5396) knots 0 0 0 0 1 1 1 1
  spline S390 degree 3 poles (242.4906, -168.5396) (242.0144, -169.0423) (241.5646, -169.7567) (241.4588, -170.1271) knots 0 0 0 0 1 1 1 1
  spline S391 degree 3 poles (241.4588, -170.1271) (241.3794, -170.4975) (240.956, -172.0585) (240.5327, -173.6196) knots 0 0 0 0 1 1 1 1
  line L136 (240.5327, -173.6196) -> (239.7654, -176.4771)
  line L137 (239.7654, -176.4771) -> (240.8502, -176.3183)
  spline S392 degree 3 poles (240.8502, -176.3183) (244.5015, -175.7363) (246.8827, -172.7465) (248.2056, -167.0315) knots 0 0 0 0 1 1 1 1
  spline S393 degree 3 poles (248.2056, -167.0315) (249.3169, -162.1896) (248.576, -158.75) (246.036, -156.9244) knots 0 0 0 0 1 1 1 1
  spline S394 degree 3 poles (246.036, -156.9244) (242.57, -154.3844) (240.1094, -156.5275) (237.3313, -164.4915) knots 0 0 0 0 1 1 1 1
  spline S395 degree 3 poles (237.3313, -164.4915) (236.3523, -167.2696) (235.929, -167.8252) (235.3469, -167.0579) knots 0 0 0 0 1 1 1 1
  spline S396 degree 3 poles (235.3469, -167.0579) (234.5002, -165.9467) (235.0823, -163.2744) (236.3523, -162.2954) knots 0 0 0 0 1 1 1 1
  spline S397 degree 3 poles (236.3523, -162.2954) (236.8815, -161.8985) (237.199, -161.1313) (237.8604, -158.75) knots 0 0 0 0 1 1 1 1
  spline S398 degree 3 poles (237.8604, -158.75) (238.3102, -157.0831) (238.7335, -155.4956) (238.8129, -155.231) knots 0 0 0 0 1 1 1 1
  spline S399 degree 3 poles (238.8129, -155.231) (238.9188, -154.8606) (238.7865, -154.7813) (237.9398, -154.7813) knots 0 0 0 0 1 1 1 1
  spline S400 degree 3 poles (237.9398, -154.7813) (237.3842, -154.8077) (236.511, -154.9929) (236.0083, -155.2046) knots 0 0 0 0 1 1 1 1
  spline S401 degree 3 poles (42.5979, -182.4567) (38.735, -184.7056) (35.4542, -186.6371) (35.269, -186.7429) knots 0 0 0 0 1 1 1 1
  spline S402 degree 3 poles (35.269, -186.7429) (35.0573, -186.8752) (36.4596, -189.5475) (39.8463, -195.3948) knots 0 0 0 0 1 1 1 1
  spline S403 degree 3 poles (39.8463, -195.3948) (42.545, -200.0515) (44.8469, -203.9673) (44.9527, -204.0731) knots 0 0 0 0 1 1 1 1
  spline S404 degree 3 poles (44.9527, -204.0731) (45.0585, -204.179) (45.9317, -203.8085) (46.8842, -203.2529) knots 0 0 0 0 1 1 1 1
  line L138 (46.8842, -203.2529) -> (48.6304, -202.2475)
  line L139 (48.6304, -202.2475) -> (45.376, -196.6383)
  line L140 (45.376, -196.6383) -> (42.1217, -191.0292)
  line L141 (42.1217, -191.0292) -> (42.9419, -190.5265)
  spline S405 degree 3 poles (42.9419, -190.5265) (43.4181, -190.2619) (45.6935, -188.939) (48.0219, -187.5896) knots 0 0 0 0 1 1 1 1
  spline S406 degree 3 poles (48.0219, -187.5896) (50.3502, -186.2402) (52.5198, -184.9967) (52.8373, -184.785) knots 0 0 0 0 1 1 1 1
  spline S407 degree 3 poles (52.8373, -184.785) (53.3929, -184.441) (53.3929, -184.4146) (51.6467, -181.3719) knots 0 0 0 0 1 1 1 1
  spline S408 degree 3 poles (51.6467, -181.3719) (50.6677, -179.705) (49.821, -178.3292) (49.7417, -178.3556) knots 0 0 0 0 1 1 1 1
  spline S409 degree 3 poles (49.7417, -178.3556) (49.6623, -178.3556) (46.4608, -180.2077) (42.5979, -182.4567) knots 0 0 0 0 1 1 1 1
  spline S410 degree 3 poles (228.0708, -179.7315) (226.3246, -180.2077) (225.1604, -181.0279) (223.3613, -182.9594) knots 0 0 0 0 1 1 1 1
  spline S411 degree 3 poles (223.3613, -182.9594) (221.3769, -185.076) (219.7365, -187.8277) (218.731, -190.7381) knots 0 0 0 0 1 1 1 1
  spline S412 degree 3 poles (218.731, -190.7381) (218.0696, -192.6696) (217.9638, -193.2781) (218.0696, -194.9715) knots 0 0 0 0 1 1 1 1
  spline S413 degree 3 poles (218.0696, -194.9715) (218.149, -196.2944) (218.3871, -197.3527) (218.7575, -198.0406) knots 0 0 0 0 1 1 1 1
  spline S414 degree 3 poles (218.7575, -198.0406) (219.9746, -200.4219) (223.0967, -202.5121) (225.9013, -202.856) knots 0 0 0 0 1 1 1 1
  spline S415 degree 3 poles (225.9013, -202.856) (229.4467, -203.2794) (233.1244, -200.6865) (236.0877, -195.6594) knots 0 0 0 0 1 1 1 1
  spline S416 degree 3 poles (236.0877, -195.6594) (239.051, -190.6058) (239.4479, -185.8963) (237.1196, -183.1181) knots 0 0 0 0 1 1 1 1
  line L142 (237.1196, -183.1181) -> (236.4052, -182.245)
  line L143 (236.4052, -182.245) -> (234.5002, -185.4994)
  spline S417 degree 3 poles (234.5002, -185.4994) (232.9127, -188.2246) (232.6481, -188.8331) (232.8598, -189.3623) knots 0 0 0 0 1 1 1 1
  spline S418 degree 3 poles (232.8598, -189.3623) (233.6006, -191.3202) (232.066, -194.5217) (229.87, -195.6858) knots 0 0 0 0 1 1 1 1
  spline S419 degree 3 poles (229.87, -195.6858) (228.0444, -196.6383) (225.3456, -195.7388) (224.2079, -193.7808) knots 0 0 0 0 1 1 1 1
  spline S420 degree 3 poles (224.2079, -193.7808) (223.4142, -192.4315) (223.4142, -191.2673) (224.2079, -189.574) knots 0 0 0 0 1 1 1 1
  spline S421 degree 3 poles (224.2079, -189.574) (224.9752, -187.96) (226.0865, -186.8752) (227.4358, -186.399) knots 0 0 0 0 1 1 1 1
  spline S422 degree 3 poles (227.4358, -186.399) (228.3619, -186.1079) (228.6529, -185.7375) (230.2933, -182.9858) knots 0 0 0 0 1 1 1 1
  spline S423 degree 3 poles (230.2933, -182.9858) (231.2988, -181.2925) (232.0396, -179.8373) (231.9867, -179.7579) knots 0 0 0 0 1 1 1 1
  spline S424 degree 3 poles (231.9867, -179.7579) (231.6692, -179.4404) (229.1556, -179.414) (228.0708, -179.7315) knots 0 0 0 0 1 1 1 1
  line L144 (56.224, -204.8933) -> (50.1385, -210.7935)
  line L145 (50.1385, -210.7935) -> (57.4146, -218.2548)
  line L146 (57.4146, -218.2548) -> (64.6642, -225.716)
  line L147 (64.6642, -225.716) -> (66.0665, -224.3138)
  spline S425 degree 3 poles (66.0665, -224.3138) (66.8338, -223.5465) (67.4688, -222.8321) (67.4688, -222.6733) knots 0 0 0 0 1 1 1 1
  spline S426 degree 3 poles (67.4688, -222.6733) (67.4688, -222.541) (65.3785, -220.345) (62.8385, -217.7785) knots 0 0 0 0 1 1 1 1
  line L148 (62.8385, -217.7785) -> (58.2083, -213.0954)
  line L149 (58.2083, -213.0954) -> (59.2138, -212.1165)
  line L150 (59.2138, -212.1165) -> (60.1927, -211.1375)
  line L151 (60.1927, -211.1375) -> (63.9498, -214.8946)
  line L152 (63.9498, -214.8946) -> (67.7333, -218.6781)
  line L153 (67.7333, -218.6781) -> (68.8446, -217.5404)
  line L154 (68.8446, -217.5404) -> (69.9823, -216.4292)
  line L155 (69.9823, -216.4292) -> (66.1988, -212.6456)
  line L156 (66.1988, -212.6456) -> (62.4417, -208.8621)
  line L157 (62.4417, -208.8621) -> (63.4735, -207.8567)
  line L158 (63.4735, -207.8567) -> (64.5054, -206.8513)
  line L159 (64.5054, -206.8513) -> (68.7917, -211.2433)
  spline S427 degree 3 poles (68.7917, -211.2433) (71.1729, -213.651) (73.2367, -215.6354) (73.3954, -215.6354) knots 0 0 0 0 1 1 1 1
  spline S428 degree 3 poles (73.3954, -215.6354) (73.5806, -215.6354) (74.295, -215.0533) (75.0094, -214.3125) knots 0 0 0 0 1 1 1 1
  line L160 (75.0094, -214.3125) -> (76.3058, -212.9896)
  line L161 (76.3058, -212.9896) -> (75.274, -211.8783)
  spline S429 degree 3 poles (75.274, -211.8783) (73.3425, -209.7881) (62.574, -198.9667) (62.4417, -198.9667) knots 0 0 0 0 1 1 1 1
  spline S430 degree 3 poles (62.4417, -198.9667) (62.3623, -198.9667) (59.5842, -201.639) (56.224, -204.8933) knots 0 0 0 0 1 1 1 1
  spline S431 degree 3 poles (208.9415, -203.0677) (207.6979, -204.4171) (206.6131, -205.6342) (206.5867, -205.74) knots 0 0 0 0 1 1 1 1
  spline S432 degree 3 poles (206.5867, -205.74) (206.5338, -205.8723) (208.8356, -208.1213) (211.6667, -210.7142) knots 0 0 0 0 1 1 1 1
  spline S433 degree 3 poles (211.6667, -210.7142) (214.4977, -213.3335) (217.3288, -215.9265) (217.9373, -216.5085) knots 0 0 0 0 1 1 1 1
  line L162 (217.9373, -216.5085) -> (219.0221, -217.5669)
  line L163 (219.0221, -217.5669) -> (220.6096, -215.8735)
  spline S434 degree 3 poles (220.6096, -215.8735) (221.4563, -214.9475) (222.541, -213.7569) (223.0173, -213.2277) knots 0 0 0 0 1 1 1 1
  line L164 (223.0173, -213.2277) -> (223.8375, -212.2488)
  line L165 (223.8375, -212.2488) -> (217.5404, -206.4279)
  line L166 (217.5404, -206.4279) -> (211.2169, -200.6071)
  line L167 (211.2169, -200.6071) -> (208.9415, -203.0677)
  line L168 (199.8398, -212.381) -> (196.9029, -214.3919)
  line L169 (196.9029, -214.3919) -> (200.2102, -219.2867)
  spline S435 degree 3 poles (200.2102, -219.2867) (202.3798, -222.4617) (203.3588, -224.1021) (203.0413, -224.0227) knots 0 0 0 0 1 1 1 1
  spline S436 degree 3 poles (203.0413, -224.0227) (199.734, -223.0173) (189.1242, -220.1333) (188.8331, -220.1333) knots 0 0 0 0 1 1 1 1
  spline S437 degree 3 poles (188.8331, -220.1333) (188.304, -220.1333) (181.901, -224.5519) (181.901, -224.9223) knots 0 0 0 0 1 1 1 1
  spline S438 degree 3 poles (181.901, -224.9223) (181.901, -225.2927) (191.0821, -238.8923) (191.3467, -238.9188) knots 0 0 0 0 1 1 1 1
  spline S439 degree 3 poles (191.3467, -238.9188) (191.7435, -238.9188) (196.9823, -235.1617) (196.9558, -234.8706) knots 0 0 0 0 1 1 1 1
  spline S440 degree 3 poles (196.9558, -234.8706) (196.9294, -234.6854) (195.5271, -232.5423) (193.8338, -230.0552) knots 0 0 0 0 1 1 1 1
  spline S441 degree 3 poles (193.8338, -230.0552) (192.1404, -227.5946) (190.8704, -225.5308) (191.0027, -225.4779) knots 0 0 0 0 1 1 1 1
  spline S442 degree 3 poles (191.0027, -225.4779) (191.135, -225.425) (194.4423, -226.2981) (198.3317, -227.4094) knots 0 0 0 0 1 1 1 1
  line L170 (198.3317, -227.4094) -> (205.4225, -229.4202)
  line L171 (205.4225, -229.4202) -> (208.8356, -227.0919)
  spline S443 degree 3 poles (208.8356, -227.0919) (210.6877, -225.8219) (212.2752, -224.7106) (212.3281, -224.6313) knots 0 0 0 0 1 1 1 1
  spline S444 degree 3 poles (212.3281, -224.6313) (212.4075, -224.5254) (206.2163, -215.265) (203.1735, -210.9523) knots 0 0 0 0 1 1 1 1
  spline S445 degree 3 poles (203.1735, -210.9523) (202.7767, -210.3702) (202.7767, -210.3702) (199.8398, -212.381) knots 0 0 0 0 1 1 1 1
  spline S446 degree 3 poles (80.354, -219.1808) (78.105, -219.8158) (75.909, -222.0383) (74.9035, -224.7635) knots 0 0 0 0 1 1 1 1
  spline S447 degree 3 poles (74.9035, -224.7635) (73.1308, -229.4996) (75.909, -234.024) (82.6823, -237.4635) knots 0 0 0 0 1 1 1 1
  spline S448 degree 3 poles (82.6823, -237.4635) (85.4604, -238.8923) (87.3919, -239.4479) (89.4821, -239.4479) knots 0 0 0 0 1 1 1 1
  spline S449 degree 3 poles (89.4821, -239.4479) (91.2812, -239.4479) (93.5831, -238.6542) (94.4298, -237.7546) knots 0 0 0 0 1 1 1 1
  line L172 (94.4298, -237.7546) -> (95.0383, -237.1196)
  line L173 (95.0383, -237.1196) -> (93.2127, -236.0613)
  spline S450 degree 3 poles (93.2127, -236.0613) (88.9794, -233.6006) (88.5031, -233.389) (88.1063, -233.6271) knots 0 0 0 0 1 1 1 1
  spline S451 degree 3 poles (88.1063, -233.6271) (87.3654, -234.1033) (85.5927, -233.9181) (84.164, -233.2038) knots 0 0 0 0 1 1 1 1
  spline S452 degree 3 poles (84.164, -233.2038) (81.5975, -231.9073) (80.5921, -229.579) (81.5975, -227.1977) knots 0 0 0 0 1 1 1 1
  spline S453 degree 3 poles (81.5975, -227.1977) (82.0738, -226.0335) (83.6613, -224.6842) (84.7725, -224.4725) knots 0 0 0 0 1 1 1 1
  spline S454 degree 3 poles (84.7725, -224.4725) (86.8892, -224.0756) (90.1171, -226.0335) (90.8315, -228.1502) knots 0 0 0 0 1 1 1 1
  spline S455 degree 3 poles (90.8315, -228.1502) (91.1754, -229.1821) (91.3871, -229.3673) (94.324, -231.0606) knots 0 0 0 0 1 1 1 1
  spline S456 degree 3 poles (94.324, -231.0606) (96.0438, -232.0396) (97.5254, -232.7804) (97.6048, -232.6746) knots 0 0 0 0 1 1 1 1
  spline S457 degree 3 poles (97.6048, -232.6746) (97.6842, -232.5952) (97.7635, -231.7221) (97.7371, -230.7431) knots 0 0 0 0 1 1 1 1
  spline S458 degree 3 poles (97.7371, -230.7431) (97.7371, -228.2825) (96.8375, -226.5098) (94.5092, -224.3138) knots 0 0 0 0 1 1 1 1
  spline S459 degree 3 poles (94.5092, -224.3138) (90.2758, -220.345) (84.111, -218.1225) (80.354, -219.1808) knots 0 0 0 0 1 1 1 1
  spline S460 degree 3 poles (103.0552, -230.7167) (102.7906, -231.7485) (102.6319, -232.6481) (102.6848, -232.701) knots 0 0 0 0 1 1 1 1
  spline S461 degree 3 poles (102.6848, -232.701) (102.7377, -232.754) (104.14, -233.1508) (105.8069, -233.6006) knots 0 0 0 0 1 1 1 1
  spline S462 degree 3 poles (105.8069, -233.6006) (107.4473, -234.0504) (108.876, -234.4473) (108.929, -234.5267) knots 0 0 0 0 1 1 1 1
  spline S463 degree 3 poles (108.929, -234.5267) (108.9819, -234.5796) (108.3204, -237.4106) (107.4473, -240.7973) knots 0 0 0 0 1 1 1 1
  spline S464 degree 3 poles (107.4473, -240.7973) (106.5742, -244.184) (105.9127, -247.015) (105.9392, -247.0679) knots 0 0 0 0 1 1 1 1
  spline S465 degree 3 poles (105.9392, -247.0679) (105.9921, -247.1208) (107.5531, -247.5442) (109.3788, -248.0469) knots 0 0 0 0 1 1 1 1
  spline S466 degree 3 poles (109.3788, -248.0469) (112.3421, -248.8406) (112.7125, -248.8935) (112.8183, -248.4967) knots 0 0 0 0 1 1 1 1
  spline S467 degree 3 poles (112.8183, -248.4967) (112.8977, -248.2321) (113.6121, -245.4275) (114.4588, -242.226) knots 0 0 0 0 1 1 1 1
  spline S468 degree 3 poles (114.4588, -242.226) (115.279, -239.0246) (115.9933, -236.3788) (116.0198, -236.3258) knots 0 0 0 0 1 1 1 1
  spline S469 degree 3 poles (116.0198, -236.3258) (116.0727, -236.2729) (117.4485, -236.6169) (119.089, -237.0402) knots 0 0 0 0 1 1 1 1
  spline S470 degree 3 poles (119.089, -237.0402) (120.7558, -237.49) (122.2375, -237.8604) (122.3963, -237.8604) knots 0 0 0 0 1 1 1 1
  spline S471 degree 3 poles (122.3963, -237.8604) (122.6608, -237.8604) (123.6927, -234.1827) (123.481, -233.971) knots 0 0 0 0 1 1 1 1
  spline S472 degree 3 poles (123.481, -233.971) (123.3488, -233.8652) (104.1929, -228.8646) (103.8225, -228.8646) knots 0 0 0 0 1 1 1 1
  spline S473 degree 3 poles (103.8225, -228.8646) (103.6373, -228.8646) (103.2933, -229.7113) (103.0552, -230.7167) knots 0 0 0 0 1 1 1 1
  spline S474 degree 3 poles (168.1692, -229.2879) (158.5648, -231.431) (154.5167, -237.199) (158.0092, -243.7606) knots 0 0 0 0 1 1 1 1
  spline S475 degree 3 poles (158.0092, -243.7606) (160.0994, -247.65) (164.1475, -248.8142) (170.2329, -247.2531) knots 0 0 0 0 1 1 1 1
  spline S476 degree 3 poles (170.2329, -247.2531) (177.0327, -245.5333) (180.7104, -242.1731) (180.7104, -237.7017) knots 0 0 0 0 1 1 1 1
  spline S477 degree 3 poles (180.7104, -237.7017) (180.7104, -234.3415) (178.8848, -231.14) (176.1067, -229.7377) knots 0 0 0 0 1 1 1 1
  spline S478 degree 3 poles (176.1067, -229.7377) (174.4133, -228.8646) (170.9738, -228.6529) (168.1692, -229.2879) knots 0 0 0 0 1 1 1 1
  spline S479 degree 3 poles (171.7675, -234.5531) (173.5667, -235.9025) (174.1752, -238.7865) (173.064, -240.6121) knots 0 0 0 0 1 1 1 1
  spline S480 degree 3 poles (173.064, -240.6121) (171.794, -242.6758) (167.8252, -243.6019) (165.8673, -242.279) knots 0 0 0 0 1 1 1 1
  spline S481 degree 3 poles (165.8673, -242.279) (164.7825, -241.5646) (163.7771, -239.686) (163.7771, -238.3896) knots 0 0 0 0 1 1 1 1
  spline S482 degree 3 poles (163.7771, -238.3896) (163.8035, -235.8496) (166.4494, -233.7594) (169.4656, -233.9446) knots 0 0 0 0 1 1 1 1
  spline S483 degree 3 poles (169.4656, -233.9446) (170.524, -233.9975) (171.3177, -234.2092) (171.7675, -234.5531) knots 0 0 0 0 1 1 1 1
  spline S484 degree 3 poles (128.2171, -234.606) (127.7408, -234.7383) (127.7408, -235.1088) (127.8467, -243.1521) knots 0 0 0 0 1 1 1 1
  spline S485 degree 3 poles (127.8467, -243.1521) (127.8996, -247.8088) (128.0054, -251.6452) (128.0583, -251.6981) knots 0 0 0 0 1 1 1 1
  spline S486 degree 3 poles (128.0583, -251.6981) (128.1377, -251.7775) (129.7517, -251.7775) (131.6567, -251.6981) knots 0 0 0 0 1 1 1 1
  line L174 (131.6567, -251.6981) -> (135.1492, -251.5394)
  line L175 (135.1492, -251.5394) -> (135.0963, -249.1317)
  line L176 (135.0963, -249.1317) -> (135.0698, -246.724)
  line L177 (135.0698, -246.724) -> (138.43, -246.724)
  spline S487 degree 3 poles (138.43, -246.724) (142.3723, -246.724) (142.9544, -246.9885) (143.7746, -249.1317) knots 0 0 0 0 1 1 1 1
  spline S488 degree 3 poles (143.7746, -249.1317) (144.0392, -249.846) (144.3567, -250.6927) (144.489, -251.0102) knots 0 0 0 0 1 1 1 1
  spline S489 degree 3 poles (144.489, -251.0102) (144.7006, -251.5923) (144.8329, -251.6188) (147.8756, -251.6188) knots 0 0 0 0 1 1 1 1
  spline S490 degree 3 poles (147.8756, -251.6188) (149.6219, -251.6188) (151.1035, -251.5129) (151.1829, -251.3806) knots 0 0 0 0 1 1 1 1
  spline S491 degree 3 poles (151.1829, -251.3806) (151.3681, -251.116) (150.6538, -247.8088) (150.2569, -247.0944) knots 0 0 0 0 1 1 1 1
  spline S492 degree 3 poles (150.2569, -247.0944) (150.1246, -246.8563) (149.6219, -246.38) (149.0927, -246.0625) knots 0 0 0 0 1 1 1 1
  line L178 (149.0927, -246.0625) -> (148.1667, -245.5069)
  line L179 (148.1667, -245.5069) -> (149.3044, -244.6602)
  spline S493 degree 3 poles (149.3044, -244.6602) (150.7596, -243.549) (151.3417, -242.3319) (151.3417, -240.5063) knots 0 0 0 0 1 1 1 1
  spline S494 degree 3 poles (151.3417, -240.5063) (151.3152, -237.6752) (150.1246, -236.1671) (147.029, -235.1352) knots 0 0 0 0 1 1 1 1
  spline S495 degree 3 poles (147.029, -235.1352) (145.5473, -234.6325) (144.6213, -234.5796) (137.0542, -234.5267) knots 0 0 0 0 1 1 1 1
  spline S496 degree 3 poles (137.0542, -234.5267) (132.4769, -234.5002) (128.5081, -234.5267) (128.2171, -234.606) knots 0 0 0 0 1 1 1 1
  spline S497 degree 3 poles (143.6423, -239.2892) (144.0392, -239.6596) (144.1979, -240.0565) (144.145, -240.6121) knots 0 0 0 0 1 1 1 1
  spline S498 degree 3 poles (144.145, -240.6121) (144.0127, -241.9085) (142.875, -242.279) (138.5888, -242.4906) knots 0 0 0 0 1 1 1 1
  line L180 (138.5888, -242.4906) -> (134.9375, -242.6758)
  line L181 (134.9375, -242.6758) -> (134.9375, -240.665)
  line L182 (134.9375, -240.665) -> (134.9375, -238.6277)
  line L183 (134.9375, -238.6277) -> (139.0121, -238.7071)
  spline S499 degree 3 poles (139.0121, -238.7071) (142.6104, -238.7865) (143.1396, -238.8394) (143.6423, -239.2892) knots 0 0 0 0 1 1 1 1
extrude "Extrude1'''" add sketch "Sketch1 (4)" along normal blind 1 separate body contours S12 S13 S14 S15 S16 S17 S18 S19 S20 S21 S22 S23 S24 | S35 S36 L6 L7 S37 S38 | S70 S71 S72 S73 S74 | S155 S156 S157 S158 S159 S160 S161 S162 L116 L117 S163 S164 S165 S166 S167 S168 S169 S170 S171 S172 S173 S174 S175 S176 S177 S178 S179 S180 S181 S182 S183 S184 S185 S186 S187 S188 S189 S190 S191 S192 L118 L119 S193 S194 L120 L121 S195 S196 S197 S198 S199 S200 S201 S202 S203 S204 S205 S206 S207 S208 S209 S210 S211 S212 S213 S214 S215 S216 S217 S218 S219 S220 S221 S222 S223 S224 S225 S226 S227 S228 S229 S230 L122 L123 S231 S232 S233 S234 S235 S236 L124 L125 S237 S238 S239 S240 S241 S242 S243 S244 S245 S246 S247 S248 S249 S250 S251 S252 S253 S254 S255 S256 S257 S258 S259 S260 S261 S262 S263 S264 S265 L126 L127 S266 S267 S268 S269 S270 S271 S272 S273 S274 S275 S276 S277 S278 S279 S280 S281 S282 S283 S284 S285 S286 S287 S288 S289 S290 S291 S292 S293 S294 L128 L129 S295 L130 L131 S296 S297 S298 S299 S300 S301 S302 S303 S304 S305 | S315 S316 S317 S318 S319 | S479 S480 S481 S482 S483 | S497 S498 L180 L181 L182 L183 S499 makes body 4 at (145.2318, 0, 35.0236) makes body 5 at (33.5175, 0, 143.7726) makes body 6 at (139.6603, 0, 144.3357) makes body 7 at (192.7456, 0, 46.136) makes body 8 at (137.5128, 0, 239.9418) makes body 9 at (171.3729, 0, 237.7605) makes body 10 at (219.7765, 0, 77.6876) in component "_Logo v2"
scale "Scale1" factor 0.15 about (146.8967, 0, 139.2502) bodies 7 4 10 8 9 6 5 in component "_Logo v2"